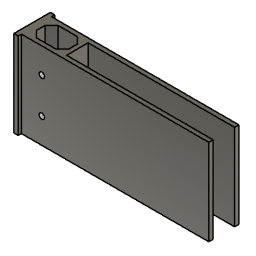
IRIV Box Camera Mount v1 (Autodesk Fusion 360 design; units mm, degrees)
Autodesk Fusion 360 part; units mm, degrees
sketch "Sketch1" plane through (0, 0, 0) normal (0, 0, 1) x (1, 0, 0)
  line L0 (0, 0) -> (70, 0)
  line L1 (70, 14) -> (0, 14)
  line L2 (0, 0) -> (2, 0)
  line L3 (2, 2) -> (70, 2)
  line L4 (70, 12) -> (2, 12)
  line L5 (2, 12) -> (2, 2)
  line L6 (70, 0) -> (70, 2)
  line L7 (70, 12) -> (70, 14)
  line L8 (0, 0) -> (-17, 0)
  line L9 (0, 14) -> (-17, 14)
  line L10 (-17, 15.5) -> (-19, 15.5)
  line L11 (-19, 15.5) -> (-19, -1.5)
  line L12 (-19, -1.5) -> (-17, -1.5)
  line L13 (-3, 12) -> (-12, 12)
  line L14 (-15, 9) -> (-15, 5)
  line L15 (-12, 2) -> (-3, 2)
  line L16 (-15, 9) -> (-12, 12)
  line L17 (-3, 12) -> (0, 9)
  line L18 (0, 5) -> (-3, 2)
  line L19 (-12, 2) -> (-15, 5)
  line L20 (-17, -1.5) -> (-17, 0)
  line L21 (-17, 14) -> (-17, 15.5)
  line L22 (-17, -1.5) -> (-17, 0)
  line L23 (-17, 14) -> (-17, 15.5)
  line L24 (0, 9) -> (0, 5)
  dimension "d1" = 70
  dimension "d2" = 14
  dimension "d3" = 2
  dimension "d4" = 2
  dimension "d6" = 17
  dimension "d8" = 1.5
  dimension "d9" = 17
  dimension "d10" = 2
  dimension "d11" = 17
  constraint horizontal L0
  constraint vertical L6
  constraint horizontal L1
  constraint coincident L0.start L2.start
  constraint horizontal L3
  constraint horizontal L4
  constraint vertical L5
  constraint coincident L4.start L6
  constraint collinear L6 L7
  constraint perpendicular L8 L20
  constraint coincident L9.end L20
  constraint perpendicular L9 L20
  constraint horizontal L10
  constraint vertical L11
  constraint horizontal L12
  constraint vertical L22
  constraint horizontal L13
  constraint vertical L14
  constraint horizontal L15
  constraint collinear L20 L21
  constraint collinear L22 L23
  measures "d1" distance of L0.start L0.end
  measures "d2" distance of L0.start L1.end
  measures "d3" distance of L0.start L2.end
  measures "d4" distance of L2.end L3.start
  measures "d6" distance of L0.start L8.end
  measures "d8" distance of L8.end L12.end
  measures "d9" distance of L12.end L10.start
  measures "d10" distance of L10.start L10.end
  measures "d11" distance of L10.start L12.end
extrude "Extrude1" add sketch "Sketch1" along normal blind 40
sketch "Sketch2" plane through (-19, 0, 0) normal (-1, 0, 0) x (0, -1, 0)
  line L0 (-15.5, 0) -> (1.5, 0)
  line L1 (1.5, 0) -> (1.5, 40)
  line L2 (1.5, 40) -> (-15.5, 40)
  line L3 (-15.5, 40) -> (-15.5, 0)
  line L4 (-7, 0) -> (-7, 40)
  line L5 (-7, 20) -> (-7, 28.25)
  line L6 (-7, 20) -> (-7, 11.75)
  circle A0 centre (-7, 11.75) radius 1.5
  circle A1 centre (-7, 28.25) radius 1.5
  dimension "d23" = 8.25
  dimension "d24" = 8.25
  dimension "d25" = 3
  dimension "d26" = 3
  constraint midpoint L0 L4.start
  constraint midpoint L2 L4.end
  constraint midpoint L4 L5.start
  constraint perpendicular L0 L5
  constraint parallel L4 L6
  constraint coincident L6.end A0.centre
  constraint coincident L5.end A1.centre
  measures "d23" distance of L5.start L5.end
  measures "d24" distance of L5.start L6.end
  measures "d25" diameter of A0
  measures "d26" diameter of A1
sketch "Sketch4" plane through (0, 14, 0) normal (0, 1, 0) x (-1, 0, 0)
  line L0 (-70, 0) -> (17, 0)
  line L1 (17, 0) -> (17, 40)
  line L2 (17, 40) -> (-70, 40)
  line L3 (-70, 40) -> (-70, 0)
  line L4 (17, 20) -> (7.5, 20)
  line L5 (7.5, 20) -> (7.5, 11.75)
  line L6 (7.5, 20) -> (7.5, 28.25)
  circle A0 centre (7.5, 11.75) radius 1.5
  circle A1 centre (7.5, 28.25) radius 1.5
  dimension "d27" = 9.5
  dimension "d28" = 8.25
  dimension "d29" = 8.25
  dimension "d30" = 3
  dimension "d31" = 3
  constraint midpoint L1 L4.start
  constraint perpendicular L1 L4
  constraint perpendicular L4 L5
  constraint perpendicular L4 L6
  constraint coincident L5.end A0.centre
  constraint coincident L6.end A1.centre
  measures "d27" distance of L4.start L4.end
  measures "d28" distance of L4.end L5.end
  measures "d29" distance of L4.end L6.end
  measures "d30" diameter of A0
  measures "d31" diameter of A1
sketch "Sketch5" plane through (0, 0, 0) normal (0, -1, 0) x (1, 0, 0)
  line L0 (-17, 0) -> (70, 0)
  line L1 (70, 0) -> (70, 40)
  line L2 (70, 40) -> (-17, 40)
  line L3 (-17, 40) -> (-17, 0)
  line L4 (-17, 20) -> (-7.5, 20)
  line L5 (-7.5, 20) -> (-7.5, 28.25)
  line L6 (-7.5, 20) -> (-7.5, 11.75)
  circle A0 centre (-7.5, 28.25) radius 1.5
  circle A1 centre (-7.5, 11.75) radius 1.5
  dimension "d32" = 9.5
  dimension "d33" = 8.25
  dimension "d34" = 8.25
  dimension "d35" = 3
  dimension "d36" = 3
  constraint midpoint L3 L4.start
  constraint perpendicular L3 L4
  constraint perpendicular L4 L5
  constraint perpendicular L4 L6
  constraint coincident L5.end A0.centre
  constraint coincident L6.end A1.centre
  measures "d32" distance of L4.start L4.end
  measures "d33" distance of L4.end L5.end
  measures "d34" distance of L4.end L6.end
  measures "d35" diameter of A0
  measures "d36" diameter of A1
extrude "Extrude2" cut sketch "Sketch2" against normal blind 4 contours L4 L6 A0 | L4 L6 A0 | L4 L5 A1 | L4 L5 A1
extrude "Extrude3" cut sketch "Sketch5" against normal blind 4 contours A0 | A1
extrude "Extrude4" cut sketch "Sketch4" against normal blind 4 contours A0 | A1
thread "Thread1" "ISO Metric profile 3.0 M3x0.5 6H" major diameter 3.086 minor diameter 2.529 pitch 0.5 angle 60 resizes the face on face at (-17.6667, 5.5075, 28.3994)
thread "Thread2" "ISO Metric profile 3.0 M3x0.5 6H" major diameter 3.086 minor diameter 2.529 pitch 0.5 angle 60 resizes the face on face at (-16.3333, 5.5019, 11.6752)
thread "Thread3" "ISO Metric profile 3.0 M3x0.5 6H" major diameter 3.086 minor diameter 2.529 pitch 0.5 angle 60 resizes the face on face at (-8.9925, 13.3333, 28.1006) on face at (-8.9925, 13.3333, 11.6006)
thread "Thread4" "ISO Metric profile 3.0 M3x0.5 6H" major diameter 3.086 minor diameter 2.529 pitch 0.5 angle 60 resizes the face on face at (-8.9925, 1.3333, 28.1006)
thread "Thread5" "ISO Metric profile 3.0 M3x0.5 6H" major diameter 3.086 minor diameter 2.529 pitch 0.5 angle 60 resizes the face on face at (-6.0075, 0.6667, 11.6006)
